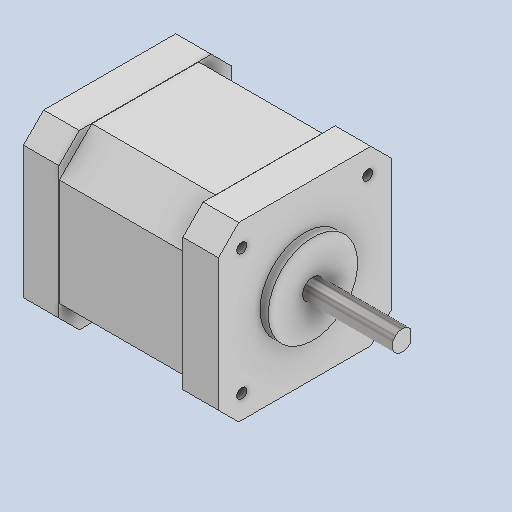
# Autodesk Inventor part: HCMUTE-CDT23-OP_STEP-42
Saved by Autodesk Inventor 2023 (Build 270158000, 158)
## iProperties
Created: 2023-11-14
Part Number: HCMUTE-CDT23-OP_STEP-42
Material: Generic
Document SubType Name: Modeling
Designer: havie
Density: 1 g/cm^3
Appearance: Default
Author: havie
Autodesk Inventor part; units mm, degrees
ref_plane "YZ Plane" through (0, 0, 0) normal (1, 0, 0) x (0, 1, 0)
ref_plane "XZ Plane" through (0, 0, 0) normal (0, 1, 0) x (-1, 0, 0)
sketch "Sketch1" plane through (0, 0, 0) normal (1, 0, 0) x (0, 1, 0)
  line L0 (21.25, 21.25) -> (-21.25, 21.25)
  line L1 (-21.25, 21.25) -> (-21.25, -21.25)
  line L2 (-21.25, -21.25) -> (21.25, -21.25)
  line L3 (21.25, -21.25) -> (21.25, 21.25)
  line L4 (21.25, 21.25) -> (-21.25, -21.25) construction
  line L5 (-21.25, 21.25) -> (21.25, -21.25) construction
  point P0 (0, 0)
  dimension "d0" = 42.5
  dimension "d1" = 42.5
  constraints: 12 end point, 2 midpoint, 2 parallel, 1 horizontal, 1 perpendicular
  measures "d0" distance of L0.end L1.end
  measures "d1" distance of L1.end L2.end
extrude "Extrusion1" add sketch "Sketch1" along normal blind 8.75
chamfer "Chamfer1" distance 5 angle 45 4 edges at (4.375, 21.25, 21.25) (4.375, 21.25, -21.25) (4.375, -21.25, 21.25) (4.375, -21.25, -21.25)
sketch "Sketch2" plane through (8.75, 0, 0) normal (1, 0, 0) x (0, 0, -1)
  line L0 (21.15, -21.15) -> (-21.15, -21.15)
  line L1 (-21.15, -21.15) -> (-21.15, 21.15)
  line L2 (-21.15, 21.15) -> (21.15, 21.15)
  line L3 (21.15, 21.15) -> (21.15, -21.15)
  line L4 (21.15, -21.15) -> (-21.15, 21.15) construction
  line L5 (-21.15, -21.15) -> (21.15, 21.15) construction
  point P0 (0, 0)
  dimension "d7" = 42.3
  dimension "d8" = 42.3
  constraints: 12 end point, 2 midpoint, 2 parallel, 1 horizontal, 1 perpendicular
  measures "d7" distance of L2.end L0.start
  measures "d8" distance of L1.end L2.end
extrude "Extrusion2" add sketch "Sketch2" along normal blind 30.5
chamfer "Chamfer2" distance 8 angle 45 4 edges at (24, 21.15, 21.15) (24, 21.15, -21.15) (24, -21.15, 21.15) (24, -21.15, -21.15)
ref_plane "Work Plane1" through (24, 0, 0) normal (1, 0, 0) x (0, 0, -1)
mirror "Mirror1" about plane through (24, 0, 0) normal (1, 0, 0) of "Extrusion1"
chamfer "Chamfer3" distance 5 angle 45 4 edges at (43.625, 21.25, -21.25) (43.625, -21.25, -21.25) (43.625, -21.25, 21.25) (43.625, 21.25, 21.25)
sketch "Sketch3" plane through (48, -16.25, 21.25) normal (1, 0, 0) x (0, 0, -1)
  point P0 (21.25, 16.25)
  point P1 (36.75, 31.75)
  point P2 (36.75, 0.75)
  point P3 (5.75, 0.75)
  point P4 (5.75, 31.75)
  dimension "d17" = 31
  dimension "d18" = 31
  dimension "d19" = 15.5
  dimension "d20" = 15.5
  constraints: 2 horizontal alignment, 2 vertical alignment
  measures "d17" distance of point (5.75, 31.75) point (36.75, 31.75)
  measures "d18" distance of point (36.75, 31.75) point (36.75, 0.75)
  measures "d19" horizontal distance of point (21.25, 16.25) point (36.75, 31.75)
  measures "d20" horizontal distance of point (5.75, 31.75) point (21.25, 16.25)
hole "Hole1" at (48, 15.5, -15.5) at (48, -15.5, -15.5) at (48, -15.5, 15.5) at (48, 15.5, 15.5) direction (-1, 0, 0) diameter 2.459 depth 18 tip angle 118 thread size "M3x0.5" class "6H" standard "ISO Metric profile"
sketch "Sketch4" plane through (48, -16.25, 21.25) normal (1, 0, 0) x (0, 0, -1)
  circle A0 centre (21.25, 16.25) radius 11
  dimension "d28" = 22
  constraints: 1 centre point, 1 coincident
  measures "d28" diameter of A0
extrude "Extrusion3" add sketch "Sketch4" along normal blind 2
sketch "Sketch5" plane through (50, 0, 0) normal (1, 0, 0) x (0, 0, -1)
  circle A0 centre (0, 0) radius 2.5
  dimension "d31" = 5
  constraints: 1 centre point, 1 coincident
  measures "d31" diameter of A0
extrude "Extrusion4" add sketch "Sketch5" along normal blind 22
sketch "Sketch6" plane through (72, 0, 0) normal (1, 0, 0) x (0, 0, -1)
  circle A0 centre (0, 0) radius 2.5 projected
  line L0 (2, 1.5) -> (2, -1.5)
  point P0 (2, 0)
  dimension "d34" = 2
  constraints: 2 end point, 2 point on circle, 1 midpoint, 1 vertical
  measures "d34" distance of point (0, 0) point (2, 0)
extrude "Extrusion5" cut sketch "Sketch6" against normal blind 20 contours A0 L0 picked at (2.0912, -0.3466)
equation "\"d1\" = d0"
equation "\"d8\" = d7"
equation "\"d18\" = d17"
body "Solid1"
